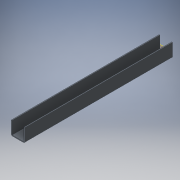
# Autodesk Inventor part: cut c channel
Saved by Autodesk Inventor 2016 (Build 200138000, 138)
## iProperties
Created: 2015-08-29
Part Number: cut c channel
Material: Generic
Description: CHANNEL - 416 MM
Document SubType Name: Modeling
Designer: PTC
Density: 1 g/cm^3
Appearance: Default
Sending System: Creo  TM  2.0  (c) 2012
PROJECT: FTC
PATTERN_NO: 6.0
PTC_MATERIAL_NAME: METAL_ALUMINIUM_5052
NIKCONFIGCOUNT: 1
KIT: TETRIX
Author: phi
Autodesk Inventor part; units mm, degrees
ref_plane "YZ Plane" through (0, 0, 0) normal (1, 0, 0) x (0, 1, 0)
ref_plane "XZ Plane" through (0, 0, 0) normal (0, 1, 0) x (-1, 0, 0)
ref_plane "XY Plane" through (0, 0, 0) normal (0, 0, 1) x (1, 0, 0)
ref_plane "FRONT" through (0, 0, 0) normal (0, 0, 1) x (1, 0, 0)
ref_plane "TOP" through (0, 0, 0) normal (0, 1, 0) x (-1, 0, 0)
ref_plane "RIGHT" through (0, 0, 0) normal (1, 0, 0) x (0, 1, 0)
ref_plane "DTM1" through (0, 0, 16) normal (0, 0, 1) x (1, 0, 0)
ref_plane "Work Plane5" through (-14, 2, 16) normal (0, 0, 1) x (1, 0, 0)
sketch "Sketch2" plane through (-14, 2, 16) normal (0, 0, 1) x (1, 0, 0)
  arc A0 (-2, 0.5) -> (0.5, -2) centre (0.5, 0.5) ccw projected
  line L0 (-2, 0.5) -> (-2, 27.5) projected
  line L1 (0, 27.5) -> (0, 0) projected
  line L2 (-2, 30) -> (-2, 27.5) projected
  line L3 (0, 27.5) -> (0, 30) projected
  line L4 (0, 30) -> (-2, 30) projected
  line L5 (0, 0) -> (28, 0) projected
  line L6 (27.5, -2) -> (0.5, -2) projected
  arc A1 (27.5, -2) -> (30, 0.5) centre (27.5, 0.5) ccw projected
  line L7 (30, 27.5) -> (30, 0.5) projected
  line L8 (28, 0) -> (28, 27.5) projected
  line L9 (28, 30) -> (28, 27.5) projected
  line L10 (30, 30) -> (28, 30) projected
  line L11 (30, 27.5) -> (30, 30) projected
  point P0 (14, -2)
extrude "Extrusion1" add sketch "Sketch2" along normal blind 352
body "Solid2"
